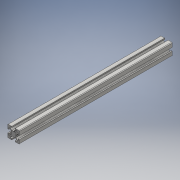
# Autodesk Inventor part: NFS5-2020-260
Saved by Autodesk Inventor 2016 (Build 200138000, 138)
## iProperties
Created: 2016-11-08
Part Number: NFS5-2020-260
Material: 一般
Document SubType Name: Modeling
Designer: 宏太
Density: 1 g/cm^3
Appearance: 既定
Author: 宏太
Autodesk Inventor part; units mm, degrees
ref_plane "YZ Plane" through (0, 0, 0) normal (1, 0, 0) x (0, 1, 0)
ref_plane "XZ Plane" through (0, 0, 0) normal (0, 1, 0) x (-1, 0, 0)
ref_plane "XY Plane" through (0, 0, 0) normal (0, 0, 1) x (1, 0, 0)
sketch "スケッチ1" plane through (0, 0, 0) normal (0, 1, 0) x (-1, 0, 0)
  line L0 (-10, 3) -> (-8, 3)
  line L1 (-8, 3) -> (-8, 6)
  line L2 (-8, 6) -> (-7.0607, 6)
  line L3 (-7.0607, 6) -> (-4, 2.9393)
  line L4 (-4, 2.9393) -> (-4, 0.6536)
  arc A0 (-4, 0.6536) -> (-3.933, 0.4036) centre (-3.5, 0.6536) ccw
  line L5 (-3.933, 0.4036) -> (-3.7, 0)
  line L6 (-3.7, 0) -> (-3.933, -0.4036)
  arc A1 (-3.933, -0.4036) -> (-3.933, -0.9036) centre (-3.5, -0.6536) ccw
  line L7 (-3.933, -0.9036) -> (-3.751, -1.2189)
  line L8 (-3.751, -1.2189) -> (-4, -2.5)
  line L9 (-4, -2.5) -> (-4, -2.9393)
  line L10 (-4, -2.9393) -> (-7.0607, -6)
  line L11 (-7.0607, -6) -> (-8, -6)
  line L12 (-8, -6) -> (-8, -3)
  line L13 (-8, -3) -> (-10, -3)
  line L14 (-10, -3) -> (-10, -9)
  arc A2 (-10, -9) -> (-9, -10) centre (-9, -9) ccw
  line L15 (-9, -10) -> (-3, -10)
  line L16 (-3, -10) -> (-3, -8)
  line L17 (-3, -8) -> (-6, -8)
  line L18 (-6, -8) -> (-6, -7.0607)
  line L19 (-6, -7.0607) -> (-2.9393, -4)
  line L20 (-2.9393, -4) -> (-0.6536, -4)
  arc A3 (-0.6536, -4) -> (-0.4036, -3.933) centre (-0.6536, -3.5) ccw
  line L21 (-0.4036, -3.933) -> (0, -3.7)
  line L22 (0, -3.7) -> (0.4036, -3.933)
  arc A4 (0.4036, -3.933) -> (0.9036, -3.933) centre (0.6536, -3.5) ccw
  line L23 (0.9036, -3.933) -> (1.2189, -3.751)
  line L24 (1.2189, -3.751) -> (2.5, -4)
  line L25 (2.5, -4) -> (2.9393, -4)
  line L26 (2.9393, -4) -> (6, -7.0607)
  line L27 (6, -7.0607) -> (6, -8)
  line L28 (6, -8) -> (3, -8)
  line L29 (3, -8) -> (3, -10)
  line L30 (3, -10) -> (9, -10)
  arc A5 (9, -10) -> (10, -9) centre (9, -9) ccw
  line L31 (10, -9) -> (10, -3)
  line L32 (10, -3) -> (8, -3)
  line L33 (8, -3) -> (8, -6)
  line L34 (8, -6) -> (7.0607, -6)
  line L35 (7.0607, -6) -> (4, -2.9393)
  line L36 (4, -2.9393) -> (4, -0.6536)
  arc A6 (4, -0.6536) -> (3.933, -0.4036) centre (3.5, -0.6536) ccw
  line L37 (3.933, -0.4036) -> (3.7, 0)
  line L38 (3.7, 0) -> (3.933, 0.4036)
  arc A7 (3.933, 0.4036) -> (3.933, 0.9036) centre (3.5, 0.6536) ccw
  line L39 (3.933, 0.9036) -> (3.751, 1.2189)
  line L40 (3.751, 1.2189) -> (4, 2.5)
  line L41 (4, 2.5) -> (4, 2.9393)
  line L42 (4, 2.9393) -> (7.0607, 6)
  line L43 (7.0607, 6) -> (8, 6)
  line L44 (8, 6) -> (8, 3)
  line L45 (8, 3) -> (10, 3)
  line L46 (10, 3) -> (10, 9)
  arc A8 (10, 9) -> (9, 10) centre (9, 9) ccw
  line L47 (9, 10) -> (3, 10)
  line L48 (3, 10) -> (3, 8)
  line L49 (3, 8) -> (6, 8)
  line L50 (6, 8) -> (6, 7.0607)
  line L51 (6, 7.0607) -> (2.9393, 4)
  line L52 (2.9393, 4) -> (0.6536, 4)
  arc A9 (0.6536, 4) -> (0.4036, 3.933) centre (0.6536, 3.5) ccw
  line L53 (0.4036, 3.933) -> (0, 3.7)
  line L54 (0, 3.7) -> (-0.4036, 3.933)
  arc A10 (-0.4036, 3.933) -> (-0.9036, 3.933) centre (-0.6536, 3.5) ccw
  line L55 (-0.9036, 3.933) -> (-1.2189, 3.751)
  line L56 (-1.2189, 3.751) -> (-2.5, 4)
  line L57 (-2.5, 4) -> (-2.9393, 4)
  line L58 (-2.9393, 4) -> (-6, 7.0607)
  line L59 (-6, 7.0607) -> (-6, 8)
  line L60 (-6, 8) -> (-3, 8)
  line L61 (-3, 8) -> (-3, 10)
  line L62 (-3, 10) -> (-9, 10)
  arc A11 (-9, 10) -> (-10, 9) centre (-9, 9) ccw
  line L63 (-10, 9) -> (-10, 3)
  point P0 (0, 0)
  constraints: 128 end point, 24 point on circle, 12 centre point
extrude "押し出し1" add sketch "スケッチ1" along normal blind 260
